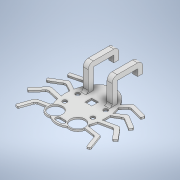
# Autodesk Inventor part: CauldronProject
Saved by Autodesk Inventor 2020 (Build 240168000, 168)
## iProperties
Created: 2021-10-31
Part Number: CauldronProject
Material: Generic
Document SubType Name: Modeling
Designer: Denil
Density: 1 g/cm^3
Appearance: Default
Author: Denil
## iProperties of the stored document _3DPrint.ipt
Created: 2021-10-31
Part Number: _3DPrint
Material: Generic
Document SubType Name: Modeling
Designer: Denil
Density: 1 g/cm^3
Appearance: Default
Author: Denil
Autodesk Inventor part; units mm, degrees
ref_plane "YZ Plane" through (0, 0, 0) normal (1, 0, 0) x (0, 1, 0)
ref_plane "Work Plane1" through (-36.5996, 16.0347, 0) normal (0, 1, 0) x (1, 0, 0)
sketch "Sketch3" plane through (-36.5996, 16.0347, 0) normal (0, 1, 0) x (1, 0, 0)
  line L0 (-29.5402, -2.779) -> (76.2931, -2.779) construction
  line L1 (76.2931, -2.779) -> (76.2931, -73.9519) construction
  line L2 (76.2931, -73.9519) -> (-29.5402, -73.9519) construction
  line L3 (-29.5402, -73.9519) -> (-29.5402, -2.779) construction
  point P0 (36.5996, 0)
  constraints: 2 other
ref_plane "Work Plane2" through (-36.5996, 16.0347, 0) normal (0, 1, 0) x (1, 0, 0)
sketch "Sketch4" plane through (-36.5996, 16.0347, 0) normal (0, 1, 0) x (1, 0, 0)
  arc A0 (19.75, -59.5) -> (19.75, -65) centre (19.75, -62.25) ccw projected
  line L0 (19.75, -59.5) -> (25.75, -59.5) projected
  arc A1 (25.75, -65) -> (25.75, -59.5) centre (25.75, -62.25) ccw projected
  line L1 (25.75, -65) -> (45.5, -65) projected
  line L2 (45.5, -65) -> (45.5, 0) projected
  line L3 (0, 0) -> (45.5, 0) projected
  line L4 (0, -65) -> (0, 0) projected
  line L5 (0, -65) -> (19.75, -65) projected
  line L6 (38.325, -45.5) -> (33.325, -45.5) projected
  line L7 (33.325, -45.5) -> (33.325, -25) projected
  line L8 (33.325, -25) -> (34.325, -26) projected
  line L9 (34.325, -26) -> (34.325, -44.5) projected
  line L10 (34.325, -44.5) -> (37.325, -44.5) projected
  line L11 (37.325, -44.5) -> (37.325, -26) projected
  line L12 (37.325, -26) -> (38.325, -25) projected
  line L13 (38.325, -25) -> (38.325, -45.5) projected
  circle A2 centre (9.675, -55) radius 8.25 projected
  circle A3 centre (35.825, -55) radius 8.25 projected
  line L14 (7.175, -25) -> (7.175, -45.5) projected
  line L15 (7.175, -25) -> (8.175, -26) projected
  line L16 (8.175, -44.5) -> (8.175, -26) projected
  line L17 (11.175, -44.5) -> (8.175, -44.5) projected
  line L18 (11.175, -26) -> (11.175, -44.5) projected
  line L19 (11.175, -26) -> (12.175, -25) projected
  line L20 (12.175, -45.5) -> (12.175, -25) projected
  line L21 (7.175, -45.5) -> (12.175, -45.5) projected
  circle A4 centre (35.5, -10) radius 2.25 projected
  circle A5 centre (10, -10) radius 2.25 projected
  line L22 (0, 0) -> (45.5, 0) projected
  line L23 (0, 0) -> (45.5, 0)
  line L24 (45.5, 0) -> (45.5, -65)
  line L25 (45.5, -65) -> (0, -65)
  line L26 (0, -65) -> (0, 0)
  circle A6 centre (35.825, -55) radius 8.4961
  circle A7 centre (9.675, -55) radius 8.25
  arc A8 (25.75, -65) -> (25.75, -59.5) centre (25.75, -62.25) ccw projected
  line L27 (25.75, -62.25) -> (19.75, -62.25) construction
  line L28 (25.75, -59.4978) -> (19.75, -59.4978)
  line L29 (19.75, -65.0022) -> (25.75, -65.0022)
  arc A9 (25.75, -65.0022) -> (25.75, -59.4978) centre (25.75, -62.25) ccw
  arc A10 (19.75, -59.4978) -> (19.75, -65.0022) centre (19.75, -62.25) ccw
  circle A11 centre (35.825, -55) radius 9.6602
  circle A12 centre (9.675, -55) radius 9.675
  line L30 (0, -65) -> (0, 0) projected
  ellipse E0 centre (22.75, -32.5) end of major axis (23.4094, -67.1502) minor radius 24.596 (34.2476, -63.3484) -> (34.5216, -63.1464) ccw
  ellipse E1 centre (22.75, -32.5) end of major axis (23.4094, -67.1502) minor radius 24.596 (43.3972, -51.7251) -> (43.5336, -51.4277) ccw
  ellipse E2 centre (22.75, -32.5) end of major axis (23.4094, -67.1502) minor radius 24.596 (12.9553, -64.1019) -> (32.9501, -64.2226) ccw
  ellipse E3 centre (22.75, -32.5) end of major axis (23.4094, -67.1502) minor radius 24.596 (44.1239, -50.0555) -> (1.5669, -49.7213) ccw
  ellipse E4 centre (22.75, -32.5) end of major axis (23.4094, -67.1502) minor radius 24.596 (2.282, -51.3386) -> (11.4397, -63.0591) ccw
  point P0 (36.5996, 0)
  point P1 (22.75, -62.25)
  constraints: 16 end point, 14 point on circle, 6 centre point, 6 tangent, 4 coincident, 3 parallel, 2 horizontal, 1 midpoint, 1 perpendicular, 20 other
extrude "Extrusion2" add sketch "Sketch4" along normal blind 2 contours A12 L21 L20 L19 L18 L17 L16 L15 L14 E3 L4 L3 L2 A11 L6 L13 L12 L11 L10 L9 L8 L7 A9 L28 A10 | A10 A12 L21 | A10 L5 E2 A12 | A9 A11 E2 L1 | L1 E2 L5 A10 L29 A9 | A12 L21 L14 L15 L16 L17 L18 L19 L20 | L21 A12 | A11 L6 | A11 L6 | L6 L7 L8 L9 L10 L11 L12 L13 A11 | E3 L4 | L2 E3 | E3 L3 | A4 | A5
sketch "Sketch5" plane through (-36.5996, 18.0347, 0) normal (0, 1, 0) x (1, 0, 0)
  ellipse E0 centre (22.75, -32.5) end of major axis (23.4094, -67.1502) minor radius 24.596 (12.9553, -64.1019) -> (32.9501, -64.2226) ccw projected
  arc A0 (32.9501, -64.2226) -> (44.1239, -50.0555) centre (35.825, -55) ccw construction
  ellipse E1 centre (22.75, -32.5) end of major axis (23.4094, -67.1502) minor radius 24.596 (44.1239, -50.0555) -> (1.5669, -49.7213) ccw projected
  arc A1 (1.5669, -49.7213) -> (12.9553, -64.1019) centre (9.675, -55) ccw construction
  line L0 (25.75, -65.0022) -> (19.75, -65.0022) construction
  arc A2 (19.75, -59.4978) -> (19.75, -65.0022) centre (19.75, -62.25) ccw construction
  line L1 (19.75, -59.4978) -> (25.75, -59.4978) construction
  arc A3 (25.75, -65.0022) -> (25.75, -59.4978) centre (25.75, -62.25) ccw construction
  circle A4 centre (9.675, -55) radius 8.25 construction
  circle A5 centre (35.825, -55) radius 8.4961 construction
  line L2 (22.75, 0) -> (22.75, -67.1503) construction
  ellipse E2 centre (22.75, -32.5) end of major axis (23.4094, -67.1502) minor radius 24.596 (12.9553, -64.1019) -> (32.9501, -64.2226) ccw projected
  line L3 (22.75, -32.5) -> (-1.8483, -32.5) construction
  ellipse E3 centre (22.75, -32.5) end of major axis (23.4094, -67.1502) minor radius 24.596 (44.1239, -50.0555) -> (1.5669, -49.7213) ccw construction
  line L4 (45.7411, -44.9978) -> (-0.2411, -44.9978) construction
  line L5 (-0.2411, -44.9978) -> (-0.2411, -65.0022) construction
  line L6 (-0.2411, -65.0022) -> (45.7411, -65.0022) construction
  line L7 (45.7411, -65.0022) -> (45.7411, -44.9978) construction
  line L8 (45.7411, -44.9978) -> (-0.2411, -65.0022) construction
  line L9 (-0.2411, -44.9978) -> (45.7411, -65.0022) construction
  line L10 (34.75, -15.2412) -> (10.75, -15.2412) construction
  line L11 (10.75, -15.2412) -> (10.75, -40.2412) construction
  line L12 (10.75, -40.2412) -> (34.75, -40.2412) construction
  line L13 (34.75, -40.2412) -> (34.75, -15.2412) construction
  line L14 (34.75, -15.2412) -> (10.75, -40.2412) construction
  line L15 (10.75, -15.2412) -> (34.75, -40.2412) construction
  line L16 (22.75, -15.2412) -> (22.75, -25.4912) construction
  line L17 (26.75, -21.4912) -> (18.75, -21.4912)
  line L18 (18.75, -21.4912) -> (18.75, -29.4912)
  line L19 (18.75, -29.4912) -> (26.75, -29.4912)
  line L20 (26.75, -29.4912) -> (26.75, -21.4912)
  line L21 (26.75, -21.4912) -> (18.75, -29.4912) construction
  line L22 (18.75, -21.4912) -> (26.75, -29.4912) construction
  line L23 (22.75, -25.4912) -> (45.4271, -25.4912) construction
  line L24 (22.75, -25.4912) -> (3.071, -25.4912) construction
  circle A6 centre (39.2405, -25.4912) radius 2.5
  circle A7 centre (6.2595, -25.4912) radius 2.5
  circle A8 centre (39.2405, -40.6364) radius 2.5
  circle A9 centre (6.2595, -40.6364) radius 2.5
  point P0 (36.5996, 0)
  point P1 (22.75, -55)
  point P2 (22.75, -27.7412)
  dimension "d28" = 24
  dimension "d29" = 25
  dimension "d30" = 10.25
  dimension "d31" = 8
  dimension "d32" = 8
  dimension "d33" = 5
  dimension "d34" = 5
  constraints: 46 end point, 7 midpoint, 6 parallel, 5 point on line, 4 centre point, 4 horizontal, 4 perpendicular, 2 symmetric about line, 1 vertical, 8 other
  measures "d28" distance of L12.end L11.end
  measures "d29" distance of L11.end L10.end
  measures "d30" distance of L16.start L16.end
  measures "d31" distance of L19.end L18.end
  measures "d32" distance of L18.end L17.end
  measures "d33" diameter of A6
  measures "d34" diameter of A8
extrude "Extrusion3" cut sketch "Sketch5" against normal blind 2
sketch "Sketch6" plane through (-36.5996, 18.0347, 0) normal (0, 1, 0) x (1, 0, 0)
  circle A0 centre (6.2595, -25.4912) radius 2.5 construction
  circle A1 centre (6.2595, -40.6364) radius 2.5 construction
  circle A2 centre (39.2405, -25.4912) radius 2.5 construction
  line L0 (18.75, -29.4912) -> (18.75, -21.4912) construction
  line L1 (18.75, -21.4912) -> (26.75, -21.4912) construction
  line L2 (26.75, -21.4912) -> (26.75, -29.4912) construction
  line L3 (26.75, -29.4912) -> (18.75, -29.4912) construction
  circle A3 centre (39.2405, -40.6364) radius 2.5 construction
  ellipse E0 centre (22.75, -32.5) end of major axis (23.4094, -67.1502) minor radius 24.596 (12.9553, -64.1019) -> (32.9501, -64.2226) ccw construction
  arc A4 (32.9501, -64.2226) -> (44.1239, -50.0555) centre (35.825, -55) ccw construction
  ellipse E1 centre (22.75, -32.5) end of major axis (23.4094, -67.1502) minor radius 24.596 (44.1239, -50.0555) -> (1.5669, -49.7213) ccw construction
  arc A5 (1.5669, -49.7213) -> (12.9553, -64.1019) centre (9.675, -55) ccw construction
  line L4 (25.75, -65.0022) -> (19.75, -65.0022) construction
  arc A6 (19.75, -59.4978) -> (19.75, -65.0022) centre (19.75, -62.25) ccw construction
  line L5 (19.75, -59.4978) -> (25.75, -59.4978) construction
  arc A7 (25.75, -65.0022) -> (25.75, -59.4978) centre (25.75, -62.25) ccw construction
  circle A8 centre (9.675, -55) radius 8.25 construction
  circle A9 centre (35.825, -55) radius 8.4961 construction
  line L6 (22.75, 0) -> (22.75, -67.1503) construction
  line L7 (39.7405, -18.5429) -> (33.7405, -18.5429)
  line L8 (33.7405, -18.5429) -> (33.7405, -12.5429)
  line L9 (33.7405, -12.5429) -> (39.7405, -12.5429)
  line L10 (39.7405, -12.5429) -> (39.7405, -18.5429)
  line L11 (39.7405, -18.5429) -> (33.7405, -12.5429) construction
  line L12 (33.7405, -18.5429) -> (39.7405, -12.5429) construction
  line L13 (5.7595, -18.5429) -> (11.7595, -18.5429)
  line L14 (11.7595, -18.5429) -> (11.7595, -12.5429)
  line L15 (11.7595, -12.5429) -> (5.7595, -12.5429)
  line L16 (5.7595, -12.5429) -> (5.7595, -18.5429)
  line L17 (5.7595, -18.5429) -> (11.7595, -12.5429) construction
  line L18 (11.7595, -18.5429) -> (5.7595, -12.5429) construction
  point P0 (36.5996, 0)
  point P1 (36.7405, -15.5429)
  point P2 (8.7595, -15.5429)
  dimension "d37" = 6
  dimension "d38" = 6
  constraints: 26 end point, 5 symmetric about line, 4 midpoint, 2 parallel, 2 perpendicular, 1 horizontal, 3 other
  measures "d37" distance of L8.end L9.end
  measures "d38" distance of L7.end L8.end
extrude "Extrusion4" add sketch "Sketch6" along normal blind 30
sketch "Sketch7" plane through (3.1408, 18.0347, 12.5429) normal (0, 0, -1) x (-1, 0, 0)
  line L0 (0, 0) -> (0, 30) projected
  line L1 (0, 30) -> (6, 30)
  line L2 (6, 30) -> (6, 24)
  line L3 (6, 24) -> (0, 24)
  line L4 (0, 24) -> (0, 30)
  line L5 (27.981, 30) -> (33.981, 30) projected
  line L6 (27.981, 30) -> (33.981, 30)
  line L7 (33.981, 30) -> (33.981, 24)
  line L8 (33.981, 24) -> (27.981, 24)
  line L9 (27.981, 24) -> (27.981, 30)
  point P0 (3.1408, -18.0347)
  point P1 (0, 24)
  dimension "d41" = 6
  dimension "d42" = 6
  dimension "d43" = 6
  dimension "d44" = 6
  constraints: 16 end point, 4 parallel, 2 horizontal, 2 perpendicular
  measures "d41" distance of L2.end L3.end
  measures "d42" distance of L1.end L2.end
  measures "d43" distance of L7.end L8.end
  measures "d44" distance of L6.end L7.end
extrude "Extrusion5" add sketch "Sketch7" along normal blind 30
fillet "Fillet1" radius 6 4 edges at (0.1408, 48.0347, 18.5429) (-27.8401, 48.0347, 18.5429) (0.1408, 48.0347, -17.4571) (-27.8401, 48.0347, -17.4571)
fillet "Fillet2" radius 3 2 edges at (-27.8401, 18.0347, 18.5429) (0.1408, 18.0347, 18.5429)
sketch "Sketch8" plane through (-30.8401, 42.0347, 12.5429) normal (0, -1, 0) x (1, 0, 0)
  line L0 (6, -30) -> (0, -30) projected
  line L1 (6, -24) -> (6, -30) projected
  line L2 (0, -30) -> (6, -30)
  line L3 (6, -30) -> (6, -24)
  line L4 (6, -24) -> (0, -24)
  line L5 (0, -24) -> (0, -30)
  line L6 (33.981, -30) -> (27.981, -30) projected
  line L7 (27.981, -24) -> (33.981, -24) projected
  line L8 (27.981, -30) -> (33.981, -30)
  line L9 (33.981, -30) -> (33.981, -24)
  line L10 (33.981, -24) -> (27.981, -24)
  line L11 (27.981, -24) -> (27.981, -30)
  point P0 (30.8401, -12.5429)
  constraints: 16 end point, 4 parallel, 2 horizontal, 2 perpendicular
extrude "Extrusion6" add sketch "Sketch8" along normal blind 8
sketch "Sketch9" plane through (-36.5996, 18.0347, 0) normal (0, 1, 0) x (1, 0, 0)
  arc A0 (1.5669, -49.7213) -> (12.9553, -64.1019) centre (9.675, -55) ccw projected
  line L0 (0.0398, -55.8772) -> (-10.5702, -57.8434)
  line L1 (-10.5702, -57.8434) -> (-16.1775, -73.7798)
  line L2 (-16.1775, -73.7798) -> (-19.9091, -72.4668)
  line L3 (-19.9091, -72.4668) -> (-13.7634, -55)
  line L4 (-13.7634, -55) -> (0.5821, -51.6948)
  line L5 (33.7405, -21.5429) -> (33.7405, -12.5429) projected
  line L6 (33.7405, -12.5429) -> (39.7405, -12.5429) projected
  line L7 (39.7405, -12.5429) -> (39.7405, -21.5429) projected
  line L8 (33.7405, -21.5429) -> (39.7405, -21.5429) projected
  line L9 (5.7595, -21.5429) -> (5.7595, -12.5429) projected
  line L10 (5.7595, -12.5429) -> (11.7595, -12.5429) projected
  line L11 (11.7595, -12.5429) -> (11.7595, -21.5429) projected
  line L12 (5.7595, -21.5429) -> (11.7595, -21.5429) projected
  circle A1 centre (6.2595, -25.4912) radius 2.5 projected
  circle A2 centre (6.2595, -40.6364) radius 2.5 projected
  circle A3 centre (39.2405, -25.4912) radius 2.5 projected
  line L13 (18.75, -29.4912) -> (18.75, -21.4912) projected
  line L14 (18.75, -21.4912) -> (26.75, -21.4912) projected
  line L15 (26.75, -21.4912) -> (26.75, -29.4912) projected
  line L16 (26.75, -29.4912) -> (18.75, -29.4912) projected
  circle A4 centre (39.2405, -40.6364) radius 2.5 projected
  ellipse E0 centre (22.75, -32.5) end of major axis (23.4094, -67.1502) minor radius 24.596 (12.9553, -64.1019) -> (32.9501, -64.2226) ccw projected
  arc A5 (32.9501, -64.2226) -> (44.1239, -50.0555) centre (35.825, -55) ccw projected
  ellipse E1 centre (22.75, -32.5) end of major axis (23.4094, -67.1502) minor radius 24.596 (44.1239, -50.0555) -> (1.5669, -49.7213) ccw projected
  arc A6 (1.5669, -49.7213) -> (12.9553, -64.1019) centre (9.675, -55) ccw projected
  line L17 (25.75, -65.0022) -> (19.75, -65.0022) projected
  arc A7 (19.75, -59.4978) -> (19.75, -65.0022) centre (19.75, -62.25) ccw projected
  line L18 (19.75, -59.4978) -> (25.75, -59.4978) projected
  arc A8 (25.75, -65.0022) -> (25.75, -59.4978) centre (25.75, -62.25) ccw projected
  circle A9 centre (9.675, -55) radius 8.25 projected
  circle A10 centre (35.825, -55) radius 8.4961 projected
  ellipse E2 centre (22.75, -32.5) end of major axis (23.4094, -67.1502) minor radius 24.596 (44.1239, -50.0555) -> (1.5669, -49.7213) ccw projected
  line L19 (-0.8272, -41.9475) -> (-15.4889, -38.6606)
  line L20 (-15.4889, -38.6606) -> (-26.9002, -51.154)
  line L21 (-26.9002, -51.154) -> (-30.072, -48.2569)
  line L22 (-30.072, -48.2569) -> (-16.8363, -33.7661)
  line L23 (-16.8363, -33.7661) -> (-1.578, -37.1867)
  line L24 (-1.578, -26.9015) -> (-11.6398, -21.4912)
  line L25 (-11.6398, -21.4912) -> (-26.2115, -30.2989)
  line L26 (-26.2115, -30.2989) -> (-28.2651, -26.9015)
  line L27 (-28.2651, -26.9015) -> (-11.6398, -16.8526)
  line L28 (-11.6398, -16.8526) -> (-0.9439, -22.7364)
  line L29 (2.1614, -13.1493) -> (-2.2055, -8.1623)
  line L30 (-2.2055, -8.1623) -> (-19.3285, -12.5042)
  line L31 (-19.3285, -12.5042) -> (-20.3681, -8.4044)
  line L32 (-20.3681, -8.4044) -> (-0.7278, -3.4243)
  line L33 (-0.7278, -3.4243) -> (4.3253, -9.1949)
  line L34 (42.1545, -11.5653) -> (49.8091, -3.1848)
  line L35 (49.8091, -3.1848) -> (68.5217, -8.165)
  line L36 (68.5217, -8.165) -> (67.3566, -12.5429)
  line L37 (67.3566, -12.5429) -> (50.9065, -8.165)
  line L38 (50.9065, -8.165) -> (44.0806, -15.6381)
  line L39 (46.5885, -24.3897) -> (57.402, -16.8526)
  line L40 (57.402, -16.8526) -> (73.9322, -26.9015)
  line L41 (73.9322, -26.9015) -> (71.5858, -30.7613)
  line L42 (71.5858, -30.7613) -> (57.402, -22.1389)
  line L43 (57.402, -22.1389) -> (47.1317, -28.3466)
  line L44 (47.1317, -37.5672) -> (64.4939, -33.8719)
  line L45 (64.4939, -33.8719) -> (76.3915, -48.2569)
  line L46 (76.3915, -48.2569) -> (72.759, -51.2613)
  line L47 (72.759, -51.2613) -> (62.3371, -38.6606)
  line L48 (62.3371, -38.6606) -> (46.4891, -42.0336)
  arc A11 (32.9501, -64.2226) -> (44.1239, -50.0555) centre (35.825, -55) ccw projected
  line L49 (44.9879, -51.9403) -> (61.8323, -54.4987)
  line L50 (61.8323, -54.4987) -> (68.5908, -72.6524)
  line L51 (68.5908, -72.6524) -> (64.9256, -74.0169)
  line L52 (64.9256, -74.0169) -> (58.9232, -57.8939)
  line L53 (58.9232, -57.8939) -> (45.4196, -56.1243)
  point P0 (36.5996, 0)
  constraints: 80 end point, 16 perpendicular, 6 parallel, 4 point on circle, 4 point on line, 15 other
extrude "Extrusion7" add sketch "Sketch9" against normal blind 2 contours A0 L0 L1 L2 L3 L4 | L19 L20 L21 L22 L23 E1 | L24 L25 L26 L27 L28 E1 | A5 L49 L50 L51 L52 L53 | L29 L30 L31 L32 L33 E1 | L34 L35 L36 L37 L38 E1 | E1 L44 L45 L46 L47 L48 | L39 L40 L41 L42 L43 E1
fillet "Fillet3" radius 3 15 edges at (-48.2394, 17.0347, 21.4912) (-48.2394, 17.0347, 16.8526) (-37.3275, 17.0347, 3.4243) (-38.8052, 17.0347, 8.1623) (-53.4359, 17.0347, 33.7661) (-52.0885, 17.0347, 38.6606) (-50.363, 17.0347, 55) (-47.1699, 17.0347, 57.8434) (22.3235, 17.0347, 57.8939) (25.7374, 17.0347, 38.6606) (27.8942, 17.0347, 33.8719) (20.8023, 17.0347, 16.8526) (20.8023, 17.0347, 22.1389) (13.2094, 17.0347, 3.1848) (14.3068, 17.0347, 8.165)
fillet "Fillet4" radius 1 14 edges at (31.9221, 17.0347, 8.165) (30.7569, 17.0347, 12.5429) (37.3326, 17.0347, 26.9015) (36.1594, 17.0347, 51.2613) (31.9911, 17.0347, 72.6524) (28.3259, 17.0347, 74.0169) (-52.7771, 17.0347, 73.7798) (-56.5088, 17.0347, 72.4668) (-63.4998, 17.0347, 51.154) (-66.6716, 17.0347, 48.2569) (-62.8112, 17.0347, 30.2989) (-64.8647, 17.0347, 26.9015) (-55.9282, 17.0347, 12.5042) (-56.9677, 17.0347, 8.4044)
body "Solid1"
body "Solid2"
